socle_toit (Autodesk Fusion 360 design; units mm, degrees)
Autodesk Fusion 360 part; units mm, degrees
sketch "Esquisse1" plane through (0, 0, 0) normal (0, 0, 1) x (1, 0, 0)
  line L0 (11.4929, 18.2859) -> (20.6929, 18.2859)
  line L1 (20.6929, 18.2859) -> (20.6929, 9.0859)
  line L2 (20.6929, 9.0859) -> (11.4929, 9.0859)
  line L3 (11.4929, 9.0859) -> (11.4929, 18.2859)
  line L4 (10.0929, 19.6859) -> (22.0929, 19.6859)
  line L5 (22.0929, 19.6859) -> (22.0929, 7.6859)
  line L6 (22.0929, 7.6859) -> (10.0929, 7.6859)
  line L7 (10.0929, 7.6859) -> (10.0929, 19.6859)
  dimension "d1" = 9.2
  dimension "d2" = 9.2
  dimension "d3" = 12
  dimension "d4" = 12
  dimension "d5" = 1.4
  dimension "d6" = 1.4
  constraint horizontal L0
  constraint vertical L1
  constraint horizontal L2
  constraint vertical L3
  constraint horizontal L4
  constraint vertical L5
  constraint horizontal L6
  constraint vertical L7
  measures "d1" distance of L0.start L0.end
  measures "d2" distance of L0.end L1.end
  measures "d3" distance of L4.start L4.end
  measures "d4" distance of L4.start L6.end
  measures "d5" distance of L0 L4
  measures "d6" distance of L1 L5
extrude "Extrusion1" add sketch "Esquisse1" along normal blind 25
